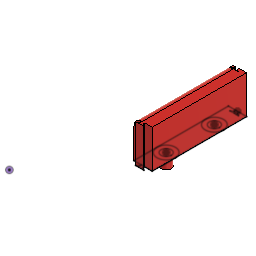
Zid teren Dreapta (Autodesk Fusion 360 design; units mm, degrees)
part number: 2026-06-02-22-21-58-545
Autodesk Fusion 360 part; units mm, degrees
sketch "Poarta Dreapta Sus" plane through (0, 0, 0) normal (0, 0, 1) x (1, 0, 0)
  line L0 (39.3447, 42.5803) -> (39.3447, 41.5803)
  line L1 (40.8447, 40.5803) -> (39.3447, 41.5803)
  line L2 (40.8447, 40.5803) -> (35.8447, 40.5803)
  line L3 (37.3447, 41.5803) -> (35.8447, 40.5803)
  line L4 (37.3447, 42.5803) -> (37.3447, 41.5803)
  circle A0 centre (38.3447, 56.5803) radius 3
  circle A1 centre (38.3447, 56.5803) radius 5.5
  circle A2 centre (38.3447, 85.7526) radius 5.5
  circle A3 centre (38.3447, 85.7526) radius 3
  line L5 (43.8447, 99.7526) -> (32.8447, 99.7526)
  line L6 (43.8447, 99.7526) -> (43.8447, 42.5803)
  line L7 (32.8447, 99.7526) -> (32.8447, 42.5803)
  line L8 (43.8447, 42.5803) -> (32.8447, 42.5803)
  line L9 (39.3447, 99.7526) -> (39.3447, 98.7526)
  line L10 (37.3447, 99.7526) -> (37.3447, 98.7526)
  line L11 (40.8447, 97.7526) -> (35.8447, 97.7526)
  line L12 (38.3447, 99.7526) -> (38.3447, 97.7526) construction
  line L13 (39.3447, 98.7526) -> (40.8447, 97.7526)
  line L14 (37.3447, 98.7526) -> (35.8447, 97.7526)
  point P0 (38.3447, 99.7526)
  dimension "d718" = 1
  dimension "d719" = 1
  dimension "d720" = 2
  dimension "d721" = 2.5
  dimension "d722" = 6
  dimension "d723" = 57.1723
  dimension "d724" = 5
  dimension "d725" = 32.8447
  dimension "d726" = 42.5803
  dimension "d727" = 2
  dimension "d728" = 3
  dimension "d729" = 14
  dimension "d730" = 43.1723
  dimension "d731" = 1
  dimension "d732" = 1
  dimension "d733" = 5
  dimension "d734" = 2
  constraint perpendicular L7 L8
  constraint midpoint L5 P0
  constraint coincident L5 L9.start
  constraint perpendicular L5 L9
  constraint tangent A1 L6
  constraint tangent A1 L7
  constraint tangent A2 L6
  constraint tangent A2 L7
  constraint concentric A0 A1
  constraint concentric A2 A3
  constraint perpendicular L5 L7
  constraint perpendicular L6 L8
  constraint parallel L0 L4
  constraint collinear L0 L9
  constraint coincident L0.start L8
  constraint coincident L4.start L8
  constraint vertical L0
  constraint horizontal L2
  constraint equal A0 A3
  constraint equal L0 L4
  constraint equal L0 L9
  constraint coincident L5 L10.start
  constraint perpendicular L5 L10
  constraint horizontal L11
  constraint coincident P0 L12.start
  constraint coincident L11 L12.end
  constraint perpendicular L11 L12
  constraint midpoint L11 L12.end
  measures "d718" distance of L9.start L9.end
  measures "d719" distance of P0 L9
  measures "d720" distance of L0.start L4.start
  measures "d721" distance of A0 A1
  measures "d722" diameter of A0
  measures "d723" distance of L5 L8
  measures "d724" horizontal distance of L1.start L2.end
  measures "d725" distance of origin L7
  measures "d726" distance of origin L8
  measures "d727" distance of L2 L8
  measures "d728" distance of L2.end L7
  measures "d729" distance of A0.centre L8
  measures "d730" distance of A2.centre L8
  measures "d731" distance of L10.start L10.end
  measures "d732" distance of P0 L10
  measures "d733" distance of L11.start L11.end
  measures "d734" distance of P0 L11
extrude "Extrude1" add sketch "Poarta Dreapta Sus" along normal blind 23 contours A1 L6 L7 L8 | L0 L1 L2 L3 L4 L8 | A1 | A1 A2 L6 L7 | A2 | A2 L5 L6 L7 L9 L10 L11 L13 L14
extrude "Extrude2" add sketch "Poarta Dreapta Sus" along normal blind 18 from surface at 5 contours A3
extrude "Extrude3" add sketch "Poarta Dreapta Sus" along normal blind 23 contours A0
extrude "Extrude4" add sketch "Poarta Dreapta Sus" against normal blind 7 contours A0
fillet "Fillet1" radius 5 2 edges at (32.8447, 71.1664, 23) (32.8447, 71.1664, 23)
